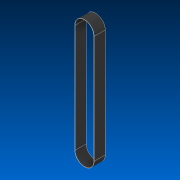
# Autodesk Inventor part: 1_16 Thick x 2 Wide Urethane Flat Belting (10 Long)(217-6002)
Saved by Autodesk Inventor 2022 (Build 260153000, 153)
## iProperties
Created: 2022-01-09
Part Number: 1_16 Thick x 2 Wide Urethane Flat Belting (10 Long)(217-6002)
Material: Rubber
Document SubType Name: Modeling
Designer: omard
Density: 0.93 g/cm^3
Appearance: Rubber - Black
Author: omard
Autodesk Inventor part; units mm, degrees
ref_plane "YZ Plane" through (0, 0, 0) normal (1, 0, 0) x (0, 1, 0)
ref_plane "XZ Plane" through (0, 0, 0) normal (0, 1, 0) x (-1, 0, 0)
ref_plane "XY Plane" through (0, 0, 0) normal (0, 0, 1) x (1, 0, 0)
sketch "Sketch1" plane through (0, 0, 0) normal (0, 0, 1) x (1, 0, 0)
  line L0 (0, 247.65) -> (0, -247.65) construction
  line L1 (-44.45, 247.65) -> (-44.45, -247.65)
  line L2 (44.45, -247.65) -> (44.45, 247.65)
  arc A0 (44.45, 247.65) -> (-44.45, 247.65) centre (0, 247.65) ccw
  arc A1 (-44.45, -247.65) -> (44.45, -247.65) centre (0, -247.65) ccw
  line L3 (-42.8625, -247.65) -> (-42.8625, 247.65)
  arc A2 (42.8625, 247.65) -> (-42.8625, 247.65) centre (0, 247.65) ccw
  line L4 (42.8625, 247.65) -> (42.8625, -247.65)
  arc A3 (-42.8625, -247.65) -> (42.8625, -247.65) centre (0, -247.65) ccw
  point P0 (0, 0)
  dimension "d0" = 495.3
  dimension "d1" = 44.45
  dimension "d2" = 1.5875
  constraints: 12 end point, 8 point on circle, 4 centre point, 4 tangent, 2 parallel, 1 midpoint, 1 vertical, 3 other
  measures "d0" distance of L0.start L0.end
  measures "d1" radius of A1
  measures "d2" distance between parallel lines of L1 L3
extrude "Extrusion1" add sketch "Sketch1" along normal mid plane 50.8
body "Solid1"
